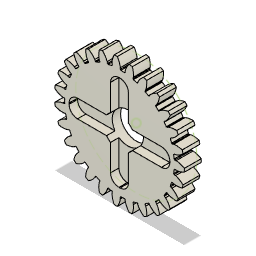
spurGearMaking (Autodesk Fusion 360 design; units mm, degrees)
description: Spur Gear; Module: 0.8; Num Teeth: 27; Pressure Angle: 20.0; Backlash: 0.00 mm
Autodesk Fusion 360 part; units mm, degrees
(part 1 of 3)
sketch "Sketch1" plane through (0, 0, 0) normal (0, 0, 1) x (1, 0, 0) in component "Spur Gear (27 teeth)"
  circle A0 centre (0, 0) radius 9.7892
  circle A1 centre (0, 0) radius 2.8
extrude "Extrude1" add sketch "Sketch1" along normal blind 3 in component "Spur Gear (27 teeth)"
sketch "Sketch2" plane through (0, 0, 0) normal (0, 0, 1) x (1, 0, 0) in component "Spur Gear (27 teeth)"
  spline S0 degree 5 poles (10.1216, -0.741) (10.1258, -0.7413) (10.1342, -0.7418) (10.1468, -0.7423) (10.1637, -0.7423) (10.1848, -0.7416) (10.2059, -0.7403) (10.2271, -0.7386) (10.2482, -0.7368) (10.2694, -0.7348) (10.2906, -0.7326) (10.3117, -0.7303) (10.3329, -0.7277) (10.3541, -0.7249) (10.3753, -0.7218) (10.3965, -0.7184) (10.4177, -0.7149) (10.4389, -0.7111) (10.4601, -0.7072) (10.4813, -0.7031) (10.5025, -0.6988) (10.5237, -0.6944) (10.5449, -0.6898) (10.5661, -0.6851) (10.5874, -0.6802) (10.6086, -0.6751) (10.6297, -0.6698) (10.6509, -0.6645) (10.6721, -0.6589) (10.6933, -0.6532) (10.7145, -0.6474) (10.7357, -0.6415) (10.7569, -0.6353) (10.778, -0.6291) (10.7992, -0.6227) (10.8204, -0.6162) (10.8415, -0.6096) (10.8627, -0.6028) (10.8838, -0.5959) (10.9049, -0.5888) (10.926, -0.5817) (10.9472, -0.5744) (10.9683, -0.5669) (10.9894, -0.5594) (11.0105, -0.5517) (11.0315, -0.544) (11.0526, -0.536) (11.0737, -0.528) (11.0947, -0.5199) (11.1158, -0.5116) (11.1368, -0.5032) (11.1578, -0.4947) (11.1788, -0.4861) (11.1998, -0.4774) (11.2208, -0.4686) (11.2418, -0.4596) (11.2628, -0.4506) (11.2837, -0.4414) (11.3047, -0.4321) (11.3256, -0.4227) (11.3465, -0.4132) (11.3674, -0.4036) (11.3883, -0.3939) (11.4092, -0.3841) (11.43, -0.3742) (11.4509, -0.3641) (11.4717, -0.354) (11.4925, -0.3438) (11.5133, -0.3334) (11.5341, -0.323) (11.5549, -0.3124) (11.5715, -0.3039) (11.5839, -0.2975) (11.5922, -0.2931) (11.5963, -0.291) knots 0 0 0 0 0 0 0.01428571 0.02857143 0.04285714 0.05714286 0.07142857 0.08571429 0.1 0.11428571 0.12857143 0.14285714 0.15714286 0.17142857 0.18571429 0.2 0.21428571 0.22857143 0.24285714 0.25714286 0.27142857 0.28571429 0.3 0.31428571 0.32857143 0.34285714 0.35714286 0.37142857 0.38571429 0.4 0.41428571 0.42857143 0.44285714 0.45714286 0.47142857 0.48571429 0.5 0.51428571 0.52857143 0.54285714 0.55714286 0.57142857 0.58571429 0.6 0.61428571 0.62857143 0.64285714 0.65714286 0.67142857 0.68571429 0.7 0.71428571 0.72857143 0.74285714 0.75714286 0.77142857 0.78571429 0.8 0.81428571 0.82857143 0.84285714 0.85714286 0.87142857 0.88571429 0.9 0.91428571 0.92857143 0.94285714 0.95714286 0.97142857 0.98571429 1 1 1 1 1 1
  spline S1 degree 5 poles (10.1216, 0.741) (10.1258, 0.7413) (10.1342, 0.7418) (10.1468, 0.7423) (10.1637, 0.7423) (10.1848, 0.7416) (10.2059, 0.7403) (10.2271, 0.7386) (10.2482, 0.7368) (10.2694, 0.7348) (10.2906, 0.7326) (10.3117, 0.7303) (10.3329, 0.7277) (10.3541, 0.7249) (10.3753, 0.7218) (10.3965, 0.7184) (10.4177, 0.7149) (10.4389, 0.7111) (10.4601, 0.7072) (10.4813, 0.7031) (10.5025, 0.6988) (10.5237, 0.6944) (10.5449, 0.6898) (10.5661, 0.6851) (10.5874, 0.6802) (10.6086, 0.6751) (10.6297, 0.6698) (10.6509, 0.6645) (10.6721, 0.6589) (10.6933, 0.6532) (10.7145, 0.6474) (10.7357, 0.6415) (10.7569, 0.6353) (10.778, 0.6291) (10.7992, 0.6227) (10.8204, 0.6162) (10.8415, 0.6096) (10.8627, 0.6028) (10.8838, 0.5959) (10.9049, 0.5888) (10.926, 0.5817) (10.9472, 0.5744) (10.9683, 0.5669) (10.9894, 0.5594) (11.0105, 0.5517) (11.0315, 0.544) (11.0526, 0.536) (11.0737, 0.528) (11.0947, 0.5199) (11.1158, 0.5116) (11.1368, 0.5032) (11.1578, 0.4947) (11.1788, 0.4861) (11.1998, 0.4774) (11.2208, 0.4686) (11.2418, 0.4596) (11.2628, 0.4506) (11.2837, 0.4414) (11.3047, 0.4321) (11.3256, 0.4227) (11.3465, 0.4132) (11.3674, 0.4036) (11.3883, 0.3939) (11.4092, 0.3841) (11.43, 0.3742) (11.4509, 0.3641) (11.4717, 0.354) (11.4925, 0.3438) (11.5133, 0.3334) (11.5341, 0.323) (11.5549, 0.3124) (11.5715, 0.3039) (11.5839, 0.2975) (11.5922, 0.2931) (11.5963, 0.291) knots 0 0 0 0 0 0 0.01428571 0.02857143 0.04285714 0.05714286 0.07142857 0.08571429 0.1 0.11428571 0.12857143 0.14285714 0.15714286 0.17142857 0.18571429 0.2 0.21428571 0.22857143 0.24285714 0.25714286 0.27142857 0.28571429 0.3 0.31428571 0.32857143 0.34285714 0.35714286 0.37142857 0.38571429 0.4 0.41428571 0.42857143 0.44285714 0.45714286 0.47142857 0.48571429 0.5 0.51428571 0.52857143 0.54285714 0.55714286 0.57142857 0.58571429 0.6 0.61428571 0.62857143 0.64285714 0.65714286 0.67142857 0.68571429 0.7 0.71428571 0.72857143 0.74285714 0.75714286 0.77142857 0.78571429 0.8 0.81428571 0.82857143 0.84285714 0.85714286 0.87142857 0.88571429 0.9 0.91428571 0.92857143 0.94285714 0.95714286 0.97142857 0.98571429 1 1 1 1 1 1
  arc A0 (11.5963, -0.291) -> (11.5963, 0.291) centre (0, 0) ccw
  line L0 (9.7531, -0.7148) -> (10.1216, -0.741)
  line L1 (9.7531, 0.7148) -> (10.1216, 0.741)
  line L2 (9.7531, -0.7148) -> (9.7531, 0.7148)
  point P0 (10.2257, -0.7387)
  point P1 (10.3304, -0.728)
  point P2 (10.4354, -0.7117)
  point P3 (10.5407, -0.6907)
  point P4 (10.6462, -0.6656)
  point P5 (10.7518, -0.6368)
  point P6 (10.8575, -0.6044)
  point P7 (10.9633, -0.5687)
  point P8 (11.069, -0.5298)
  point P9 (11.1747, -0.4878)
  point P10 (11.2803, -0.4429)
  point P11 (11.3858, -0.395)
  point P12 (11.4912, -0.3444)
  point P13 (10.2257, 0.7387)
  point P14 (10.3304, 0.728)
  point P15 (10.4354, 0.7117)
  point P16 (10.5407, 0.6907)
  point P17 (10.6462, 0.6656)
  point P18 (10.7518, 0.6368)
  point P19 (10.8575, 0.6044)
  point P20 (10.9633, 0.5687)
  point P21 (11.069, 0.5298)
  point P22 (11.1747, 0.4878)
  point P23 (11.2803, 0.4429)
  point P24 (11.3858, 0.395)
  point P25 (11.4912, 0.3444)
extrude "Extrude2" add sketch "Sketch2" along normal blind 3 in component "Spur Gear (27 teeth)"
fillet "Fillet1" radius 0.1 2 edges at (9.763, -0.7155, 1.5) (9.763, 0.7155, 1.5) in component "Spur Gear (27 teeth)"
pattern_circular "C-Pattern1" count 27 over 360 about axis through (0, 0, 0) along (0, 0, 1) of "Extrude2", "Fillet1" in component "Spur Gear (27 teeth)"
sketch "Sketch3" plane through (0, 0, 0) normal (0, 0, 1) x (1, 0, 0) in component "Spur Gear (27 teeth)"
  circle A0 centre (0, 0) radius 10.8 construction
sketch "Sketch4" plane through (0, 0, 3) normal (0, 0, 1) x (1, 0, 0) in component "Spur Gear (27 teeth)"
  arc A0 (9.6801, -1.4577) -> (9.7553, -0.814) centre (0, 0) ccw
  arc A1 (9.8621, -0.7225) -> (9.7553, -0.814) centre (9.855, -0.8223) ccw
  line L0 (9.8621, -0.7225) -> (10.1216, -0.741)
  spline S0 degree 5 poles (10.1216, -0.741) (10.1258, -0.7413) (10.1342, -0.7418) (10.1468, -0.7423) (10.1637, -0.7423) (10.1848, -0.7416) (10.2059, -0.7403) (10.2271, -0.7386) (10.2482, -0.7368) (10.2694, -0.7348) (10.2906, -0.7326) (10.3117, -0.7303) (10.3329, -0.7277) (10.3541, -0.7249) (10.3753, -0.7218) (10.3965, -0.7184) (10.4177, -0.7149) (10.4389, -0.7111) (10.4601, -0.7072) (10.4813, -0.7031) (10.5025, -0.6988) (10.5237, -0.6944) (10.5449, -0.6898) (10.5661, -0.6851) (10.5874, -0.6802) (10.6086, -0.6751) (10.6297, -0.6698) (10.6509, -0.6645) (10.6721, -0.6589) (10.6933, -0.6532) (10.7145, -0.6474) (10.7357, -0.6415) (10.7569, -0.6353) (10.778, -0.6291) (10.7992, -0.6227) (10.8204, -0.6162) (10.8415, -0.6096) (10.8627, -0.6028) (10.8838, -0.5959) (10.9049, -0.5888) (10.926, -0.5817) (10.9472, -0.5744) (10.9683, -0.5669) (10.9894, -0.5594) (11.0105, -0.5517) (11.0315, -0.544) (11.0526, -0.536) (11.0737, -0.528) (11.0947, -0.5199) (11.1158, -0.5116) (11.1368, -0.5032) (11.1578, -0.4947) (11.1788, -0.4861) (11.1998, -0.4774) (11.2208, -0.4686) (11.2418, -0.4596) (11.2628, -0.4506) (11.2837, -0.4414) (11.3047, -0.4321) (11.3256, -0.4227) (11.3465, -0.4132) (11.3674, -0.4036) (11.3883, -0.3939) (11.4092, -0.3841) (11.43, -0.3742) (11.4509, -0.3641) (11.4717, -0.354) (11.4925, -0.3438) (11.5133, -0.3334) (11.5341, -0.323) (11.5549, -0.3124) (11.5715, -0.3039) (11.5839, -0.2975) (11.5922, -0.2931) (11.5963, -0.291) knots 0 0 0 0 0 0 0.01428571 0.02857143 0.04285714 0.05714286 0.07142857 0.08571429 0.1 0.11428571 0.12857143 0.14285714 0.15714286 0.17142857 0.18571429 0.2 0.21428571 0.22857143 0.24285714 0.25714286 0.27142857 0.28571429 0.3 0.31428571 0.32857143 0.34285714 0.35714286 0.37142857 0.38571429 0.4 0.41428571 0.42857143 0.44285714 0.45714286 0.47142857 0.48571429 0.5 0.51428571 0.52857143 0.54285714 0.55714286 0.57142857 0.58571429 0.6 0.61428571 0.62857143 0.64285714 0.65714286 0.67142857 0.68571429 0.7 0.71428571 0.72857143 0.74285714 0.75714286 0.77142857 0.78571429 0.8 0.81428571 0.82857143 0.84285714 0.85714286 0.87142857 0.88571429 0.9 0.91428571 0.92857143 0.94285714 0.95714286 0.97142857 0.98571429 1 1 1 1 1 1
  arc A2 (11.5963, -0.291) -> (11.5963, 0.291) centre (0, 0) ccw
  spline S1 degree 5 poles (11.5963, 0.291) (11.5922, 0.2931) (11.5839, 0.2975) (11.5715, 0.3039) (11.5549, 0.3124) (11.5341, 0.323) (11.5133, 0.3334) (11.4925, 0.3438) (11.4717, 0.354) (11.4509, 0.3641) (11.43, 0.3742) (11.4092, 0.3841) (11.3883, 0.3939) (11.3674, 0.4036) (11.3465, 0.4132) (11.3256, 0.4227) (11.3047, 0.4321) (11.2837, 0.4414) (11.2628, 0.4506) (11.2418, 0.4596) (11.2208, 0.4686) (11.1998, 0.4774) (11.1788, 0.4861) (11.1578, 0.4947) (11.1368, 0.5032) (11.1158, 0.5116) (11.0947, 0.5199) (11.0737, 0.528) (11.0526, 0.536) (11.0315, 0.544) (11.0105, 0.5517) (10.9894, 0.5594) (10.9683, 0.5669) (10.9472, 0.5744) (10.926, 0.5817) (10.9049, 0.5888) (10.8838, 0.5959) (10.8627, 0.6028) (10.8415, 0.6096) (10.8204, 0.6162) (10.7992, 0.6227) (10.778, 0.6291) (10.7569, 0.6353) (10.7357, 0.6415) (10.7145, 0.6474) (10.6933, 0.6532) (10.6721, 0.6589) (10.6509, 0.6645) (10.6297, 0.6698) (10.6086, 0.6751) (10.5874, 0.6802) (10.5661, 0.6851) (10.5449, 0.6898) (10.5237, 0.6944) (10.5025, 0.6988) (10.4813, 0.7031) (10.4601, 0.7072) (10.4389, 0.7111) (10.4177, 0.7149) (10.3965, 0.7184) (10.3753, 0.7218) (10.3541, 0.7249) (10.3329, 0.7277) (10.3117, 0.7303) (10.2906, 0.7326) (10.2694, 0.7348) (10.2482, 0.7368) (10.2271, 0.7386) (10.2059, 0.7403) (10.1848, 0.7416) (10.1637, 0.7423) (10.1468, 0.7423) (10.1342, 0.7418) (10.1258, 0.7413) (10.1216, 0.741) knots -1 -1 -1 -1 -1 -1 -0.98571429 -0.97142857 -0.95714286 -0.94285714 -0.92857143 -0.91428571 -0.9 -0.88571429 -0.87142857 -0.85714286 -0.84285714 -0.82857143 -0.81428571 -0.8 -0.78571429 -0.77142857 -0.75714286 -0.74285714 -0.72857143 -0.71428571 -0.7 -0.68571429 -0.67142857 -0.65714286 -0.64285714 -0.62857143 -0.61428571 -0.6 -0.58571429 -0.57142857 -0.55714286 -0.54285714 -0.52857143 -0.51428571 -0.5 -0.48571429 -0.47142857 -0.45714286 -0.44285714 -0.42857143 -0.41428571 -0.4 -0.38571429 -0.37142857 -0.35714286 -0.34285714 -0.32857143 -0.31428571 -0.3 -0.28571429 -0.27142857 -0.25714286 -0.24285714 -0.22857143 -0.21428571 -0.2 -0.18571429 -0.17142857 -0.15714286 -0.14285714 -0.12857143 -0.11428571 -0.1 -0.08571429 -0.07142857 -0.05714286 -0.04285714 -0.02857143 -0.01428571 0 0 0 0 0 0
  line L1 (10.1216, 0.741) -> (9.8621, 0.7225)
  arc A3 (9.7553, 0.814) -> (9.8621, 0.7225) centre (9.855, 0.8223) ccw
  arc A4 (9.7553, 0.814) -> (9.6801, 1.4577) centre (0, 0) ccw
  arc A5 (9.7629, 1.5713) -> (9.6801, 1.4577) centre (9.7789, 1.4726) ccw
  line L2 (9.7629, 1.5713) -> (10.0197, 1.6131)
  spline S2 degree 5 poles (10.0197, 1.6131) (10.0238, 1.6138) (10.0321, 1.6153) (10.0445, 1.6178) (10.0609, 1.6216) (10.0813, 1.6272) (10.1016, 1.6333) (10.1217, 1.6398) (10.1419, 1.6465) (10.162, 1.6533) (10.1821, 1.6603) (10.2022, 1.6674) (10.2222, 1.6748) (10.2422, 1.6825) (10.2621, 1.6904) (10.282, 1.6985) (10.3018, 1.7069) (10.3215, 1.7155) (10.3412, 1.7242) (10.3609, 1.7331) (10.3806, 1.7421) (10.4002, 1.7512) (10.4198, 1.7606) (10.4393, 1.7701) (10.4588, 1.7798) (10.4783, 1.7896) (10.4977, 1.7996) (10.5171, 1.8097) (10.5364, 1.82) (10.5557, 1.8304) (10.575, 1.841) (10.5942, 1.8517) (10.6134, 1.8625) (10.6326, 1.8734) (10.6517, 1.8845) (10.6708, 1.8957) (10.6898, 1.9071) (10.7089, 1.9186) (10.7278, 1.9302) (10.7468, 1.9419) (10.7657, 1.9537) (10.7845, 1.9657) (10.8034, 1.9778) (10.8222, 1.99) (10.8409, 2.0023) (10.8596, 2.0148) (10.8783, 2.0273) (10.897, 2.04) (10.9156, 2.0528) (10.9341, 2.0657) (10.9527, 2.0787) (10.9712, 2.0918) (10.9896, 2.105) (11.008, 2.1183) (11.0264, 2.1318) (11.0448, 2.1453) (11.0631, 2.1589) (11.0814, 2.1727) (11.0996, 2.1866) (11.1178, 2.2005) (11.136, 2.2146) (11.1541, 2.2288) (11.1722, 2.243) (11.1902, 2.2574) (11.2082, 2.2719) (11.2262, 2.2864) (11.2441, 2.3011) (11.262, 2.3159) (11.2799, 2.3307) (11.2977, 2.3457) (11.3154, 2.3607) (11.3296, 2.3729) (11.3403, 2.382) (11.3473, 2.3881) (11.3509, 2.3912) knots 0 0 0 0 0 0 0.01428571 0.02857143 0.04285714 0.05714286 0.07142857 0.08571429 0.1 0.11428571 0.12857143 0.14285714 0.15714286 0.17142857 0.18571429 0.2 0.21428571 0.22857143 0.24285714 0.25714286 0.27142857 0.28571429 0.3 0.31428571 0.32857143 0.34285714 0.35714286 0.37142857 0.38571429 0.4 0.41428571 0.42857143 0.44285714 0.45714286 0.47142857 0.48571429 0.5 0.51428571 0.52857143 0.54285714 0.55714286 0.57142857 0.58571429 0.6 0.61428571 0.62857143 0.64285714 0.65714286 0.67142857 0.68571429 0.7 0.71428571 0.72857143 0.74285714 0.75714286 0.77142857 0.78571429 0.8 0.81428571 0.82857143 0.84285714 0.85714286 0.87142857 0.88571429 0.9 0.91428571 0.92857143 0.94285714 0.95714286 0.97142857 0.98571429 1 1 1 1 1 1
  arc A6 (11.3509, 2.3912) -> (11.2167, 2.9574) centre (0, 0) ccw
  spline S3 degree 5 poles (11.2167, 2.9574) (11.2121, 2.9586) (11.2031, 2.9609) (11.1895, 2.9643) (11.1714, 2.9687) (11.1487, 2.9742) (11.1261, 2.9796) (11.1035, 2.9848) (11.0808, 2.99) (11.0582, 2.9951) (11.0356, 3) (11.013, 3.0049) (10.9905, 3.0096) (10.9679, 3.0142) (10.9454, 3.0188) (10.9228, 3.0232) (10.9003, 3.0275) (10.8778, 3.0317) (10.8553, 3.0358) (10.8328, 3.0398) (10.8103, 3.0436) (10.7878, 3.0474) (10.7654, 3.051) (10.743, 3.0546) (10.7206, 3.058) (10.6982, 3.0613) (10.6758, 3.0645) (10.6534, 3.0676) (10.6311, 3.0705) (10.6087, 3.0733) (10.5864, 3.0761) (10.5641, 3.0786) (10.5419, 3.0811) (10.5196, 3.0835) (10.4974, 3.0857) (10.4752, 3.0878) (10.453, 3.0898) (10.4308, 3.0916) (10.4087, 3.0934) (10.3866, 3.0949) (10.3645, 3.0964) (10.3424, 3.0977) (10.3204, 3.0989) (10.2984, 3.1) (10.2764, 3.1009) (10.2544, 3.1017) (10.2325, 3.1023) (10.2106, 3.1028) (10.1887, 3.1032) (10.1669, 3.1034) (10.1451, 3.1035) (10.1233, 3.1033) (10.1016, 3.1031) (10.0799, 3.1026) (10.0583, 3.102) (10.0367, 3.1013) (10.0151, 3.1004) (9.9935, 3.0993) (9.972, 3.0981) (9.9506, 3.0967) (9.9292, 3.0951) (9.9078, 3.0932) (9.8866, 3.0911) (9.8654, 3.0887) (9.8442, 3.086) (9.8231, 3.0832) (9.8021, 3.0803) (9.7811, 3.0772) (9.7601, 3.074) (9.7393, 3.0704) (9.7186, 3.0662) (9.7022, 3.0623) (9.69, 3.0589) (9.6819, 3.0565) (9.6779, 3.0553) knots -1 -1 -1 -1 -1 -1 -0.98571429 -0.97142857 -0.95714286 -0.94285714 -0.92857143 -0.91428571 -0.9 -0.88571429 -0.87142857 -0.85714286 -0.84285714 -0.82857143 -0.81428571 -0.8 -0.78571429 -0.77142857 -0.75714286 -0.74285714 -0.72857143 -0.71428571 -0.7 -0.68571429 -0.67142857 -0.65714286 -0.64285714 -0.62857143 -0.61428571 -0.6 -0.58571429 -0.57142857 -0.55714286 -0.54285714 -0.52857143 -0.51428571 -0.5 -0.48571429 -0.47142857 -0.45714286 -0.44285714 -0.42857143 -0.41428571 -0.4 -0.38571429 -0.37142857 -0.35714286 -0.34285714 -0.32857143 -0.31428571 -0.3 -0.28571429 -0.27142857 -0.25714286 -0.24285714 -0.22857143 -0.21428571 -0.2 -0.18571429 -0.17142857 -0.15714286 -0.14285714 -0.12857143 -0.11428571 -0.1 -0.08571429 -0.07142857 -0.05714286 -0.04285714 -0.02857143 -0.01428571 0 0 0 0 0 0
  line L3 (9.6779, 3.0553) -> (9.4296, 2.9774)
  arc A7 (9.3046, 3.0418) -> (9.4296, 2.9774) centre (9.3997, 3.0728) ccw
  arc A8 (9.3046, 3.0418) -> (9.083, 3.6508) centre (0, 0) ccw
  arc A9 (9.1373, 3.7804) -> (9.083, 3.6508) centre (9.1758, 3.6881) ccw
  line L4 (9.1373, 3.7804) -> (9.3776, 3.8804)
  spline S4 degree 5 poles (9.3776, 3.8804) (9.3814, 3.882) (9.3892, 3.8853) (9.4007, 3.8906) (9.4158, 3.8981) (9.4343, 3.9082) (9.4526, 3.9189) (9.4707, 3.9298) (9.4888, 3.941) (9.5068, 3.9523) (9.5248, 3.9637) (9.5427, 3.9753) (9.5604, 3.9871) (9.5781, 3.9991) (9.5957, 4.0114) (9.6131, 4.0239) (9.6304, 4.0366) (9.6477, 4.0495) (9.6649, 4.0626) (9.682, 4.0757) (9.699, 4.089) (9.716, 4.1025) (9.7329, 4.1161) (9.7497, 4.1299) (9.7665, 4.1438) (9.7831, 4.1578) (9.7997, 4.172) (9.8162, 4.1864) (9.8327, 4.2008) (9.8491, 4.2154) (9.8654, 4.2301) (9.8816, 4.2449) (9.8978, 4.2599) (9.9139, 4.275) (9.93, 4.2902) (9.946, 4.3055) (9.9619, 4.3209) (9.9777, 4.3365) (9.9935, 4.3522) (10.0093, 4.3679) (10.0249, 4.3838) (10.0405, 4.3998) (10.0561, 4.4159) (10.0715, 4.4321) (10.0869, 4.4484) (10.1023, 4.4649) (10.1176, 4.4814) (10.1328, 4.498) (10.1479, 4.5147) (10.163, 4.5316) (10.1781, 4.5485) (10.193, 4.5655) (10.208, 4.5826) (10.2228, 4.5998) (10.2376, 4.6172) (10.2523, 4.6346) (10.267, 4.6521) (10.2816, 4.6697) (10.2961, 4.6874) (10.3106, 4.7051) (10.3251, 4.723) (10.3394, 4.741) (10.3537, 4.759) (10.368, 4.7772) (10.3822, 4.7954) (10.3963, 4.8137) (10.4104, 4.8321) (10.4244, 4.8506) (10.4383, 4.8692) (10.4522, 4.8879) (10.466, 4.9066) (10.477, 4.9217) (10.4853, 4.933) (10.4907, 4.9406) (10.4935, 4.9444) knots 0 0 0 0 0 0 0.01428571 0.02857143 0.04285714 0.05714286 0.07142857 0.08571429 0.1 0.11428571 0.12857143 0.14285714 0.15714286 0.17142857 0.18571429 0.2 0.21428571 0.22857143 0.24285714 0.25714286 0.27142857 0.28571429 0.3 0.31428571 0.32857143 0.34285714 0.35714286 0.37142857 0.38571429 0.4 0.41428571 0.42857143 0.44285714 0.45714286 0.47142857 0.48571429 0.5 0.51428571 0.52857143 0.54285714 0.55714286 0.57142857 0.58571429 0.6 0.61428571 0.62857143 0.64285714 0.65714286 0.67142857 0.68571429 0.7 0.71428571 0.72857143 0.74285714 0.75714286 0.77142857 0.78571429 0.8 0.81428571 0.82857143 0.84285714 0.85714286 0.87142857 0.88571429 0.9 0.91428571 0.92857143 0.94285714 0.95714286 0.97142857 0.98571429 1 1 1 1 1 1
  arc A10 (10.4935, 4.9444) -> (10.2323, 5.4645) centre (0, 0) ccw
  spline S5 degree 5 poles (10.2323, 5.4645) (10.2276, 5.4645) (10.2183, 5.4647) (10.2043, 5.4648) (10.1856, 5.465) (10.1623, 5.4651) (10.139, 5.4651) (10.1158, 5.465) (10.0926, 5.4648) (10.0694, 5.4645) (10.0463, 5.4642) (10.0232, 5.4637) (10.0002, 5.4631) (9.9771, 5.4624) (9.9541, 5.4616) (9.9312, 5.4607) (9.9083, 5.4597) (9.8854, 5.4586) (9.8626, 5.4574) (9.8398, 5.4561) (9.817, 5.4546) (9.7943, 5.4531) (9.7716, 5.4515) (9.749, 5.4497) (9.7264, 5.4479) (9.7038, 5.4459) (9.6813, 5.4439) (9.6588, 5.4417) (9.6364, 5.4394) (9.614, 5.437) (9.5917, 5.4345) (9.5694, 5.4319) (9.5472, 5.4292) (9.525, 5.4263) (9.5028, 5.4234) (9.4807, 5.4203) (9.4587, 5.4171) (9.4367, 5.4138) (9.4148, 5.4104) (9.3929, 5.4068) (9.371, 5.4032) (9.3493, 5.3994) (9.3275, 5.3954) (9.3059, 5.3914) (9.2843, 5.3872) (9.2627, 5.3829) (9.2413, 5.3785) (9.2198, 5.3739) (9.1985, 5.3692) (9.1772, 5.3644) (9.1559, 5.3594) (9.1348, 5.3543) (9.1137, 5.349) (9.0927, 5.3436) (9.0718, 5.338) (9.0509, 5.3323) (9.0301, 5.3264) (9.0094, 5.3204) (8.9888, 5.3143) (8.9682, 5.308) (8.9478, 5.3015) (8.9274, 5.2947) (8.9072, 5.2877) (8.8872, 5.2805) (8.8672, 5.2731) (8.8473, 5.2655) (8.8275, 5.2578) (8.8077, 5.25) (8.7881, 5.242) (8.7687, 5.2336) (8.7495, 5.2248) (8.7344, 5.2172) (8.7233, 5.2111) (8.716, 5.2069) (8.7124, 5.2048) knots -1 -1 -1 -1 -1 -1 -0.98571429 -0.97142857 -0.95714286 -0.94285714 -0.92857143 -0.91428571 -0.9 -0.88571429 -0.87142857 -0.85714286 -0.84285714 -0.82857143 -0.81428571 -0.8 -0.78571429 -0.77142857 -0.75714286 -0.74285714 -0.72857143 -0.71428571 -0.7 -0.68571429 -0.67142857 -0.65714286 -0.64285714 -0.62857143 -0.61428571 -0.6 -0.58571429 -0.57142857 -0.55714286 -0.54285714 -0.52857143 -0.51428571 -0.5 -0.48571429 -0.47142857 -0.45714286 -0.44285714 -0.42857143 -0.41428571 -0.4 -0.38571429 -0.37142857 -0.35714286 -0.34285714 -0.32857143 -0.31428571 -0.3 -0.28571429 -0.27142857 -0.25714286 -0.24285714 -0.22857143 -0.21428571 -0.2 -0.18571429 -0.17142857 -0.15714286 -0.14285714 -0.12857143 -0.11428571 -0.1 -0.08571429 -0.07142857 -0.05714286 -0.04285714 -0.02857143 -0.01428571 0 0 0 0 0 0
  line L5 (8.7124, 5.2048) -> (8.4888, 5.0718)
  arc A11 (8.3523, 5.1056) -> (8.4888, 5.0718) centre (8.4377, 5.1577) ccw
  arc A12 (8.3523, 5.1056) -> (7.9962, 5.647) centre (0, 0) ccw
  arc A13 (8.0192, 5.7857) -> (7.9962, 5.647) centre (8.0779, 5.7047) ccw
  line L6 (8.0192, 5.7857) -> (8.2299, 5.9384)
  spline S6 degree 5 poles (8.2299, 5.9384) (8.2333, 5.9408) (8.2401, 5.9459) (8.2501, 5.9536) (8.263, 5.9645) (8.2787, 5.9786) (8.294, 5.9932) (8.3092, 6.008) (8.3242, 6.023) (8.3391, 6.0382) (8.3539, 6.0534) (8.3687, 6.0688) (8.3833, 6.0844) (8.3977, 6.1002) (8.4119, 6.1162) (8.426, 6.1324) (8.4399, 6.1488) (8.4537, 6.1653) (8.4675, 6.1819) (8.4811, 6.1987) (8.4946, 6.2156) (8.508, 6.2326) (8.5213, 6.2497) (8.5345, 6.267) (8.5476, 6.2844) (8.5606, 6.3019) (8.5734, 6.3195) (8.5862, 6.3373) (8.5989, 6.3552) (8.6115, 6.3731) (8.6239, 6.3912) (8.6363, 6.4094) (8.6486, 6.4277) (8.6608, 6.4461) (8.6729, 6.4646) (8.685, 6.4831) (8.6969, 6.5018) (8.7087, 6.5206) (8.7205, 6.5395) (8.7321, 6.5585) (8.7437, 6.5776) (8.7552, 6.5967) (8.7666, 6.616) (8.7779, 6.6353) (8.7892, 6.6547) (8.8003, 6.6742) (8.8114, 6.6939) (8.8223, 6.7135) (8.8332, 6.7333) (8.844, 6.7532) (8.8548, 6.7731) (8.8654, 6.7931) (8.876, 6.8132) (8.8865, 6.8334) (8.8968, 6.8537) (8.9072, 6.874) (8.9174, 6.8944) (8.9276, 6.9149) (8.9376, 6.9355) (8.9476, 6.9561) (8.9575, 6.9768) (8.9674, 6.9976) (8.9771, 7.0185) (8.9868, 7.0394) (8.9964, 7.0604) (9.0059, 7.0815) (9.0154, 7.1027) (9.0247, 7.1239) (9.034, 7.1452) (9.0432, 7.1666) (9.0524, 7.188) (9.0596, 7.2052) (9.065, 7.2181) (9.0686, 7.2268) (9.0704, 7.2311) knots 0 0 0 0 0 0 0.01428571 0.02857143 0.04285714 0.05714286 0.07142857 0.08571429 0.1 0.11428571 0.12857143 0.14285714 0.15714286 0.17142857 0.18571429 0.2 0.21428571 0.22857143 0.24285714 0.25714286 0.27142857 0.28571429 0.3 0.31428571 0.32857143 0.34285714 0.35714286 0.37142857 0.38571429 0.4 0.41428571 0.42857143 0.44285714 0.45714286 0.47142857 0.48571429 0.5 0.51428571 0.52857143 0.54285714 0.55714286 0.57142857 0.58571429 0.6 0.61428571 0.62857143 0.64285714 0.65714286 0.67142857 0.68571429 0.7 0.71428571 0.72857143 0.74285714 0.75714286 0.77142857 0.78571429 0.8 0.81428571 0.82857143 0.84285714 0.85714286 0.87142857 0.88571429 0.9 0.91428571 0.92857143 0.94285714 0.95714286 0.97142857 0.98571429 1 1 1 1 1 1
  arc A14 (9.0704, 7.2311) -> (8.6963, 7.6769) centre (0, 0) ccw
  spline S7 degree 5 poles (8.6963, 7.6769) (8.6917, 7.6759) (8.6826, 7.6739) (8.6689, 7.6708) (8.6507, 7.6666) (8.628, 7.6614) (8.6054, 7.656) (8.5828, 7.6506) (8.5603, 7.645) (8.5378, 7.6394) (8.5154, 7.6337) (8.493, 7.6279) (8.4707, 7.622) (8.4485, 7.616) (8.4263, 7.6099) (8.4042, 7.6038) (8.3821, 7.5975) (8.3601, 7.5912) (8.3382, 7.5847) (8.3163, 7.5782) (8.2945, 7.5716) (8.2727, 7.5648) (8.251, 7.558) (8.2294, 7.5511) (8.2078, 7.5441) (8.1863, 7.537) (8.1649, 7.5298) (8.1435, 7.5225) (8.1222, 7.5151) (8.101, 7.5076) (8.0799, 7.5) (8.0588, 7.4924) (8.0378, 7.4846) (8.0168, 7.4767) (7.996, 7.4687) (7.9752, 7.4606) (7.9545, 7.4524) (7.9338, 7.4441) (7.9133, 7.4357) (7.8928, 7.4272) (7.8724, 7.4186) (7.8521, 7.4099) (7.8318, 7.4011) (7.8117, 7.3921) (7.7916, 7.3831) (7.7717, 7.3739) (7.7518, 7.3647) (7.732, 7.3553) (7.7123, 7.3458) (7.6927, 7.3362) (7.6732, 7.3265) (7.6538, 7.3166) (7.6345, 7.3066) (7.6153, 7.2965) (7.5962, 7.2862) (7.5772, 7.2758) (7.5584, 7.2653) (7.5396, 7.2547) (7.5209, 7.244) (7.5024, 7.2331) (7.484, 7.2221) (7.4657, 7.2108) (7.4477, 7.1994) (7.4298, 7.1877) (7.4121, 7.1759) (7.3945, 7.1639) (7.377, 7.1518) (7.3596, 7.1397) (7.3423, 7.1273) (7.3253, 7.1148) (7.3087, 7.1018) (7.2958, 7.0909) (7.2864, 7.0824) (7.2803, 7.0766) (7.2773, 7.0737) knots -1 -1 -1 -1 -1 -1 -0.98571429 -0.97142857 -0.95714286 -0.94285714 -0.92857143 -0.91428571 -0.9 -0.88571429 -0.87142857 -0.85714286 -0.84285714 -0.82857143 -0.81428571 -0.8 -0.78571429 -0.77142857 -0.75714286 -0.74285714 -0.72857143 -0.71428571 -0.7 -0.68571429 -0.67142857 -0.65714286 -0.64285714 -0.62857143 -0.61428571 -0.6 -0.58571429 -0.57142857 -0.55714286 -0.54285714 -0.52857143 -0.51428571 -0.5 -0.48571429 -0.47142857 -0.45714286 -0.44285714 -0.42857143 -0.41428571 -0.4 -0.38571429 -0.37142857 -0.35714286 -0.34285714 -0.32857143 -0.31428571 -0.3 -0.28571429 -0.27142857 -0.25714286 -0.24285714 -0.22857143 -0.21428571 -0.2 -0.18571429 -0.17142857 -0.15714286 -0.14285714 -0.12857143 -0.11428571 -0.1 -0.08571429 -0.07142857 -0.05714286 -0.04285714 -0.02857143 -0.01428571 0 0 0 0 0 0
  line L7 (7.2773, 7.0737) -> (7.0903, 6.8927)
  arc A15 (6.9498, 6.8941) -> (7.0903, 6.8927) centre (7.0208, 6.9646) ccw
  arc A16 (6.9498, 6.8941) -> (6.4784, 7.3389) centre (0, 0) ccw
  arc A17 (6.4688, 7.4791) -> (6.4784, 7.3389) centre (6.5445, 7.4139) ccw
  line L8 (6.4688, 7.4791) -> (6.6386, 7.6763)
  spline S8 degree 5 poles (6.6386, 7.6763) (6.6413, 7.6794) (6.6468, 7.6859) (6.6547, 7.6958) (6.6648, 7.7093) (6.6768, 7.7266) (6.6884, 7.7443) (6.6997, 7.7623) (6.7108, 7.7804) (6.7218, 7.7985) (6.7327, 7.8168) (6.7435, 7.8352) (6.7541, 7.8537) (6.7645, 7.8724) (6.7747, 7.8912) (6.7846, 7.9103) (6.7944, 7.9294) (6.8041, 7.9487) (6.8136, 7.968) (6.823, 7.9875) (6.8322, 8.007) (6.8413, 8.0267) (6.8503, 8.0464) (6.8592, 8.0662) (6.8679, 8.0862) (6.8765, 8.1062) (6.8849, 8.1264) (6.8933, 8.1466) (6.9015, 8.1669) (6.9096, 8.1873) (6.9176, 8.2077) (6.9254, 8.2283) (6.9332, 8.2489) (6.9408, 8.2696) (6.9483, 8.2904) (6.9557, 8.3113) (6.963, 8.3322) (6.9702, 8.3532) (6.9773, 8.3743) (6.9843, 8.3955) (6.9911, 8.4167) (6.9979, 8.438) (7.0046, 8.4594) (7.0111, 8.4808) (7.0176, 8.5023) (7.0239, 8.5238) (7.0301, 8.5455) (7.0363, 8.5671) (7.0423, 8.5889) (7.0483, 8.6107) (7.0541, 8.6326) (7.0598, 8.6545) (7.0655, 8.6765) (7.071, 8.6986) (7.0765, 8.7207) (7.0818, 8.7428) (7.0871, 8.7651) (7.0922, 8.7873) (7.0973, 8.8097) (7.1023, 8.8321) (7.1071, 8.8545) (7.1119, 8.877) (7.1166, 8.8996) (7.1212, 8.9222) (7.1257, 8.9448) (7.1301, 8.9676) (7.1344, 8.9903) (7.1386, 9.0131) (7.1427, 9.036) (7.1467, 9.0589) (7.1507, 9.0819) (7.1538, 9.1003) (7.156, 9.1141) (7.1575, 9.1233) (7.1583, 9.1279) knots 0 0 0 0 0 0 0.01428571 0.02857143 0.04285714 0.05714286 0.07142857 0.08571429 0.1 0.11428571 0.12857143 0.14285714 0.15714286 0.17142857 0.18571429 0.2 0.21428571 0.22857143 0.24285714 0.25714286 0.27142857 0.28571429 0.3 0.31428571 0.32857143 0.34285714 0.35714286 0.37142857 0.38571429 0.4 0.41428571 0.42857143 0.44285714 0.45714286 0.47142857 0.48571429 0.5 0.51428571 0.52857143 0.54285714 0.55714286 0.57142857 0.58571429 0.6 0.61428571 0.62857143 0.64285714 0.65714286 0.67142857 0.68571429 0.7 0.71428571 0.72857143 0.74285714 0.75714286 0.77142857 0.78571429 0.8 0.81428571 0.82857143 0.84285714 0.85714286 0.87142857 0.88571429 0.9 0.91428571 0.92857143 0.94285714 0.95714286 0.97142857 0.98571429 1 1 1 1 1 1
  arc A18 (7.1583, 9.1279) -> (6.6915, 9.4755) centre (0, 0) ccw
  spline S9 degree 5 poles (6.6915, 9.4755) (6.6872, 9.4734) (6.6788, 9.4694) (6.6662, 9.4632) (6.6495, 9.455) (6.6286, 9.4446) (6.6078, 9.4342) (6.5871, 9.4237) (6.5665, 9.4131) (6.5459, 9.4025) (6.5254, 9.3917) (6.505, 9.3809) (6.4846, 9.37) (6.4644, 9.3591) (6.4442, 9.3481) (6.4241, 9.337) (6.4041, 9.3258) (6.3841, 9.3145) (6.3642, 9.3032) (6.3445, 9.2918) (6.3248, 9.2803) (6.3051, 9.2687) (6.2856, 9.2571) (6.2662, 9.2454) (6.2468, 9.2336) (6.2275, 9.2217) (6.2083, 9.2098) (6.1892, 9.1978) (6.1702, 9.1857) (6.1513, 9.1735) (6.1324, 9.1612) (6.1137, 9.1489) (6.095, 9.1365) (6.0765, 9.124) (6.058, 9.1114) (6.0397, 9.0987) (6.0214, 9.086) (6.0032, 9.0731) (5.9852, 9.0602) (5.9672, 9.0472) (5.9493, 9.0342) (5.9316, 9.021) (5.9139, 9.0077) (5.8964, 8.9944) (5.879, 8.981) (5.8616, 8.9674) (5.8444, 8.9538) (5.8273, 8.9402) (5.8103, 8.9264) (5.7935, 8.9125) (5.7767, 8.8985) (5.7601, 8.8845) (5.7437, 8.8703) (5.7273, 8.856) (5.7111, 8.8416) (5.6951, 8.8272) (5.6791, 8.8126) (5.6633, 8.7979) (5.6476, 8.7832) (5.6321, 8.7683) (5.6167, 8.7533) (5.6016, 8.7382) (5.5867, 8.7228) (5.572, 8.7074) (5.5574, 8.6918) (5.5431, 8.6761) (5.5288, 8.6603) (5.5147, 8.6444) (5.5008, 8.6285) (5.4871, 8.6123) (5.4739, 8.5958) (5.4639, 8.5823) (5.4567, 8.5719) (5.4521, 8.5648) (5.4498, 8.5613) knots -1 -1 -1 -1 -1 -1 -0.98571429 -0.97142857 -0.95714286 -0.94285714 -0.92857143 -0.91428571 -0.9 -0.88571429 -0.87142857 -0.85714286 -0.84285714 -0.82857143 -0.81428571 -0.8 -0.78571429 -0.77142857 -0.75714286 -0.74285714 -0.72857143 -0.71428571 -0.7 -0.68571429 -0.67142857 -0.65714286 -0.64285714 -0.62857143 -0.61428571 -0.6 -0.58571429 -0.57142857 -0.55714286 -0.54285714 -0.52857143 -0.51428571 -0.5 -0.48571429 -0.47142857 -0.45714286 -0.44285714 -0.42857143 -0.41428571 -0.4 -0.38571429 -0.37142857 -0.35714286 -0.34285714 -0.32857143 -0.31428571 -0.3 -0.28571429 -0.27142857 -0.25714286 -0.24285714 -0.22857143 -0.21428571 -0.2 -0.18571429 -0.17142857 -0.15714286 -0.14285714 -0.12857143 -0.11428571 -0.1 -0.08571429 -0.07142857 -0.05714286 -0.04285714 -0.02857143 -0.01428571 0 0 0 0 0 0
  line L9 (5.4498, 8.5613) -> (5.3096, 8.3421)
  arc A19 (5.1726, 8.311) -> (5.3096, 8.3421) centre (5.2254, 8.3959) ccw
  arc A20 (5.1726, 8.311) -> (4.6113, 8.6351) centre (0, 0) ccw
  arc A21 (4.5696, 8.7693) -> (4.6113, 8.6351) centre (4.6584, 8.7233) ccw
  line L10 (4.5696, 8.7693) -> (4.6894, 9.0003)
  spline S10 degree 5 poles (4.6894, 9.0003) (4.6913, 9.004) (4.6951, 9.0116) (4.7005, 9.023) (4.7072, 9.0385) (4.7149, 9.0581) (4.7221, 9.078) (4.729, 9.0981) (4.7356, 9.1183) (4.7422, 9.1385) (4.7486, 9.1588) (4.7548, 9.1791) (4.7609, 9.1996) (4.7667, 9.2202) (4.7722, 9.2409) (4.7775, 9.2617) (4.7826, 9.2826) (4.7876, 9.3035) (4.7924, 9.3246) (4.797, 9.3457) (4.8015, 9.3668) (4.8059, 9.388) (4.8101, 9.4093) (4.8141, 9.4307) (4.818, 9.4521) (4.8217, 9.4736) (4.8253, 9.4951) (4.8287, 9.5167) (4.832, 9.5383) (4.8352, 9.5601) (4.8383, 9.5818) (4.8412, 9.6036) (4.844, 9.6255) (4.8466, 9.6474) (4.8491, 9.6693) (4.8515, 9.6914) (4.8538, 9.7134) (4.856, 9.7355) (4.858, 9.7577) (4.8599, 9.7799) (4.8617, 9.8021) (4.8633, 9.8244) (4.8649, 9.8467) (4.8663, 9.8691) (4.8676, 9.8915) (4.8688, 9.9139) (4.8699, 9.9364) (4.8709, 9.9589) (4.8718, 9.9815) (4.8725, 10.004) (4.8731, 10.0267) (4.8737, 10.0493) (4.8741, 10.072) (4.8744, 10.0948) (4.8746, 10.1176) (4.8747, 10.1404) (4.8747, 10.1632) (4.8746, 10.1861) (4.8743, 10.209) (4.874, 10.2319) (4.8736, 10.2549) (4.873, 10.2779) (4.8724, 10.3009) (4.8716, 10.3239) (4.8708, 10.347) (4.8698, 10.3701) (4.8688, 10.3933) (4.8676, 10.4165) (4.8663, 10.4396) (4.865, 10.4629) (4.8635, 10.4861) (4.8623, 10.5047) (4.8613, 10.5187) (4.8606, 10.528) (4.8603, 10.5327) knots 0 0 0 0 0 0 0.01428571 0.02857143 0.04285714 0.05714286 0.07142857 0.08571429 0.1 0.11428571 0.12857143 0.14285714 0.15714286 0.17142857 0.18571429 0.2 0.21428571 0.22857143 0.24285714 0.25714286 0.27142857 0.28571429 0.3 0.31428571 0.32857143 0.34285714 0.35714286 0.37142857 0.38571429 0.4 0.41428571 0.42857143 0.44285714 0.45714286 0.47142857 0.48571429 0.5 0.51428571 0.52857143 0.54285714 0.55714286 0.57142857 0.58571429 0.6 0.61428571 0.62857143 0.64285714 0.65714286 0.67142857 0.68571429 0.7 0.71428571 0.72857143 0.74285714 0.75714286 0.77142857 0.78571429 0.8 0.81428571 0.82857143 0.84285714 0.85714286 0.87142857 0.88571429 0.9 0.91428571 0.92857143 0.94285714 0.95714286 0.97142857 0.98571429 1 1 1 1 1 1
  arc A22 (4.8603, 10.5327) -> (4.3259, 10.7632) centre (0, 0) ccw
  spline S11 degree 5 poles (4.3259, 10.7632) (4.3223, 10.7603) (4.315, 10.7543) (4.3042, 10.7455) (4.2898, 10.7336) (4.2719, 10.7187) (4.254, 10.7038) (4.2363, 10.6888) (4.2187, 10.6737) (4.2011, 10.6586) (4.1836, 10.6434) (4.1663, 10.6282) (4.149, 10.6129) (4.1318, 10.5976) (4.1147, 10.5822) (4.0977, 10.5668) (4.0808, 10.5513) (4.064, 10.5357) (4.0472, 10.5201) (4.0306, 10.5045) (4.0141, 10.4887) (3.9977, 10.473) (3.9813, 10.4571) (3.9651, 10.4413) (3.949, 10.4253) (3.933, 10.4093) (3.917, 10.3933) (3.9012, 10.3772) (3.8855, 10.361) (3.8699, 10.3448) (3.8544, 10.3285) (3.839, 10.3122) (3.8237, 10.2958) (3.8086, 10.2794) (3.7935, 10.2629) (3.7786, 10.2463) (3.7637, 10.2297) (3.749, 10.213) (3.7344, 10.1963) (3.7199, 10.1795) (3.7055, 10.1626) (3.6913, 10.1457) (3.6772, 10.1288) (3.6632, 10.1117) (3.6493, 10.0947) (3.6356, 10.0775) (3.622, 10.0603) (3.6085, 10.043) (3.5952, 10.0257) (3.582, 10.0083) (3.5689, 9.9909) (3.556, 9.9734) (3.5432, 9.9558) (3.5306, 9.9381) (3.5182, 9.9204) (3.5059, 9.9026) (3.4937, 9.8847) (3.4817, 9.8668) (3.4698, 9.8489) (3.4582, 9.8308) (3.4467, 9.8127) (3.4354, 9.7944) (3.4244, 9.7761) (3.4137, 9.7577) (3.4032, 9.7391) (3.3928, 9.7205) (3.3826, 9.7019) (3.3725, 9.6832) (3.3626, 9.6645) (3.3531, 9.6456) (3.344, 9.6265) (3.3374, 9.611) (3.3328, 9.5992) (3.3299, 9.5913) (3.3285, 9.5873) knots -1 -1 -1 -1 -1 -1 -0.98571429 -0.97142857 -0.95714286 -0.94285714 -0.92857143 -0.91428571 -0.9 -0.88571429 -0.87142857 -0.85714286 -0.84285714 -0.82857143 -0.81428571 -0.8 -0.78571429 -0.77142857 -0.75714286 -0.74285714 -0.72857143 -0.71428571 -0.7 -0.68571429 -0.67142857 -0.65714286 -0.64285714 -0.62857143 -0.61428571 -0.6 -0.58571429 -0.57142857 -0.55714286 -0.54285714 -0.52857143 -0.51428571 -0.5 -0.48571429 -0.47142857 -0.45714286 -0.44285714 -0.42857143 -0.41428571 -0.4 -0.38571429 -0.37142857 -0.35714286 -0.34285714 -0.32857143 -0.31428571 -0.3 -0.28571429 -0.27142857 -0.25714286 -0.24285714 -0.22857143 -0.21428571 -0.2 -0.18571429 -0.17142857 -0.15714286 -0.14285714 -0.12857143 -0.11428571 -0.1 -0.08571429 -0.07142857 -0.05714286 -0.04285714 -0.02857143 -0.01428571 0 0 0 0 0 0
  line L11 (3.3285, 9.5873) -> (3.2427, 9.3417)
  arc A23 (3.1165, 9.2799) -> (3.2427, 9.3417) centre (3.1483, 9.3747) ccw
  arc A24 (3.1165, 9.2799) -> (2.4956, 9.4658) centre (0, 0) ccw
  arc A25 (2.4241, 9.5868) -> (2.4956, 9.4658) centre (2.5211, 9.5624) ccw
  line L12 (2.4241, 9.5868) -> (2.4874, 9.8391)
  spline S12 degree 5 poles (2.4874, 9.8391) (2.4884, 9.8432) (2.4903, 9.8514) (2.493, 9.8638) (2.496, 9.8804) (2.4989, 9.9013) (2.5013, 9.9223) (2.5033, 9.9434) (2.5052, 9.9646) (2.5069, 9.9858) (2.5084, 10.007) (2.5098, 10.0283) (2.511, 10.0496) (2.5119, 10.0709) (2.5125, 10.0923) (2.5129, 10.1138) (2.513, 10.1353) (2.513, 10.1568) (2.5128, 10.1784) (2.5124, 10.2) (2.5119, 10.2216) (2.5113, 10.2433) (2.5105, 10.265) (2.5095, 10.2867) (2.5083, 10.3084) (2.507, 10.3302) (2.5055, 10.3519) (2.5039, 10.3738) (2.5021, 10.3956) (2.5002, 10.4174) (2.4981, 10.4393) (2.4959, 10.4612) (2.4936, 10.4831) (2.4911, 10.505) (2.4885, 10.527) (2.4858, 10.549) (2.4829, 10.571) (2.4799, 10.593) (2.4768, 10.615) (2.4735, 10.637) (2.4701, 10.6591) (2.4666, 10.6811) (2.463, 10.7032) (2.4592, 10.7253) (2.4553, 10.7474) (2.4513, 10.7695) (2.4472, 10.7916) (2.4429, 10.8138) (2.4386, 10.8359) (2.4341, 10.8581) (2.4295, 10.8802) (2.4248, 10.9024) (2.4199, 10.9246) (2.415, 10.9468) (2.4099, 10.969) (2.4048, 10.9912) (2.3995, 11.0134) (2.3941, 11.0356) (2.3886, 11.0579) (2.383, 11.0801) (2.3773, 11.1024) (2.3714, 11.1246) (2.3655, 11.1469) (2.3594, 11.1691) (2.3533, 11.1914) (2.347, 11.2137) (2.3407, 11.2359) (2.3342, 11.2582) (2.3276, 11.2805) (2.3209, 11.3028) (2.3141, 11.3251) (2.3086, 11.3429) (2.3045, 11.3563) (2.3017, 11.3652) (2.3002, 11.3696) knots 0 0 0 0 0 0 0.01428571 0.02857143 0.04285714 0.05714286 0.07142857 0.08571429 0.1 0.11428571 0.12857143 0.14285714 0.15714286 0.17142857 0.18571429 0.2 0.21428571 0.22857143 0.24285714 0.25714286 0.27142857 0.28571429 0.3 0.31428571 0.32857143 0.34285714 0.35714286 0.37142857 0.38571429 0.4 0.41428571 0.42857143 0.44285714 0.45714286 0.47142857 0.48571429 0.5 0.51428571 0.52857143 0.54285714 0.55714286 0.57142857 0.58571429 0.6 0.61428571 0.62857143 0.64285714 0.65714286 0.67142857 0.68571429 0.7 0.71428571 0.72857143 0.74285714 0.75714286 0.77142857 0.78571429 0.8 0.81428571 0.82857143 0.84285714 0.85714286 0.87142857 0.88571429 0.9 0.91428571 0.92857143 0.94285714 0.95714286 0.97142857 0.98571429 1 1 1 1 1 1
  arc A26 (2.3002, 11.3696) -> (1.7271, 11.4707) centre (0, 0) ccw
  spline S13 degree 5 poles (1.7271, 11.4707) (1.7243, 11.467) (1.7186, 11.4596) (1.7101, 11.4484) (1.6988, 11.4336) (1.6848, 11.4149) (1.6709, 11.3963) (1.6571, 11.3776) (1.6434, 11.3589) (1.6298, 11.3401) (1.6163, 11.3213) (1.6029, 11.3025) (1.5896, 11.2837) (1.5764, 11.2648) (1.5633, 11.2459) (1.5504, 11.2269) (1.5375, 11.208) (1.5247, 11.1889) (1.512, 11.1699) (1.4995, 11.1508) (1.487, 11.1317) (1.4747, 11.1126) (1.4624, 11.0934) (1.4503, 11.0742) (1.4383, 11.055) (1.4264, 11.0357) (1.4146, 11.0165) (1.4029, 10.9971) (1.3914, 10.9778) (1.3799, 10.9584) (1.3686, 10.939) (1.3574, 10.9196) (1.3463, 10.9001) (1.3353, 10.8806) (1.3245, 10.8611) (1.3137, 10.8415) (1.3031, 10.8219) (1.2927, 10.8023) (1.2823, 10.7827) (1.2721, 10.763) (1.262, 10.7433) (1.252, 10.7235) (1.2422, 10.7038) (1.2325, 10.684) (1.223, 10.6642) (1.2136, 10.6443) (1.2043, 10.6244) (1.1952, 10.6045) (1.1862, 10.5846) (1.1773, 10.5646) (1.1686, 10.5446) (1.1601, 10.5246) (1.1518, 10.5045) (1.1436, 10.4844) (1.1355, 10.4643) (1.1277, 10.4442) (1.12, 10.424) (1.1124, 10.4038) (1.105, 10.3836) (1.0978, 10.3633) (1.0908, 10.343) (1.0841, 10.3227) (1.0776, 10.3023) (1.0714, 10.2819) (1.0655, 10.2614) (1.0597, 10.241) (1.054, 10.2205) (1.0485, 10.2) (1.0432, 10.1794) (1.0383, 10.1589) (1.0339, 10.1382) (1.031, 10.1216) (1.0292, 10.1091) (1.0283, 10.1007) (1.0278, 10.0965) knots -1 -1 -1 -1 -1 -1 -0.98571429 -0.97142857 -0.95714286 -0.94285714 -0.92857143 -0.91428571 -0.9 -0.88571429 -0.87142857 -0.85714286 -0.84285714 -0.82857143 -0.81428571 -0.8 -0.78571429 -0.77142857 -0.75714286 -0.74285714 -0.72857143 -0.71428571 -0.7 -0.68571429 -0.67142857 -0.65714286 -0.64285714 -0.62857143 -0.61428571 -0.6 -0.58571429 -0.57142857 -0.55714286 -0.54285714 -0.52857143 -0.51428571 -0.5 -0.48571429 -0.47142857 -0.45714286 -0.44285714 -0.42857143 -0.41428571 -0.4 -0.38571429 -0.37142857 -0.35714286 -0.34285714 -0.32857143 -0.31428571 -0.3 -0.28571429 -0.27142857 -0.25714286 -0.24285714 -0.22857143 -0.21428571 -0.2 -0.18571429 -0.17142857 -0.15714286 -0.14285714 -0.12857143 -0.11428571 -0.1 -0.08571429 -0.07142857 -0.05714286 -0.04285714 -0.02857143 -0.01428571 0 0 0 0 0 0
  line L13 (1.0278, 10.0965) -> (1.001, 9.8377)
  arc A27 (0.8924, 9.7484) -> (1.001, 9.8377) centre (0.9015, 9.848) ccw
  arc A28 (0.8924, 9.7484) -> (0.2454, 9.7861) centre (0, 0) ccw
  arc A29 (0.1479, 9.8874) -> (0.2454, 9.7861) centre (0.2479, 9.8861) ccw
  line L14 (0.1479, 9.8874) -> (0.1513, 10.1476)
  spline S14 degree 5 poles (0.1513, 10.1476) (0.1513, 10.1518) (0.1513, 10.1602) (0.151, 10.1728) (0.1501, 10.1897) (0.1481, 10.2107) (0.1456, 10.2317) (0.1427, 10.2527) (0.1396, 10.2737) (0.1364, 10.2947) (0.133, 10.3157) (0.1295, 10.3368) (0.1257, 10.3578) (0.1216, 10.3787) (0.1173, 10.3997) (0.1127, 10.4207) (0.1079, 10.4416) (0.1029, 10.4626) (0.0978, 10.4835) (0.0924, 10.5045) (0.087, 10.5254) (0.0813, 10.5463) (0.0755, 10.5672) (0.0696, 10.5881) (0.0634, 10.609) (0.0571, 10.6299) (0.0506, 10.6507) (0.044, 10.6716) (0.0373, 10.6924) (0.0304, 10.7132) (0.0233, 10.734) (0.0161, 10.7548) (0.0088, 10.7756) (0.0014, 10.7964) (-0.0062, 10.8171) (-0.014, 10.8379) (-0.0219, 10.8586) (-0.0299, 10.8793) (-0.038, 10.9) (-0.0462, 10.9207) (-0.0546, 10.9414) (-0.0631, 10.962) (-0.0718, 10.9827) (-0.0805, 11.0033) (-0.0894, 11.0239) (-0.0984, 11.0445) (-0.1075, 11.0651) (-0.1168, 11.0856) (-0.1261, 11.1062) (-0.1356, 11.1267) (-0.1452, 11.1472) (-0.1549, 11.1677) (-0.1647, 11.1882) (-0.1746, 11.2087) (-0.1847, 11.2291) (-0.1948, 11.2495) (-0.2051, 11.2699) (-0.2154, 11.2903) (-0.2259, 11.3107) (-0.2365, 11.331) (-0.2472, 11.3513) (-0.258, 11.3716) (-0.2689, 11.3919) (-0.2799, 11.4122) (-0.2911, 11.4324) (-0.3023, 11.4527) (-0.3136, 11.4729) (-0.3251, 11.4931) (-0.3366, 11.5132) (-0.3482, 11.5334) (-0.36, 11.5535) (-0.3694, 11.5696) (-0.3766, 11.5816) (-0.3814, 11.5896) (-0.3838, 11.5936) knots 0 0 0 0 0 0 0.01428571 0.02857143 0.04285714 0.05714286 0.07142857 0.08571429 0.1 0.11428571 0.12857143 0.14285714 0.15714286 0.17142857 0.18571429 0.2 0.21428571 0.22857143 0.24285714 0.25714286 0.27142857 0.28571429 0.3 0.31428571 0.32857143 0.34285714 0.35714286 0.37142857 0.38571429 0.4 0.41428571 0.42857143 0.44285714 0.45714286 0.47142857 0.48571429 0.5 0.51428571 0.52857143 0.54285714 0.55714286 0.57142857 0.58571429 0.6 0.61428571 0.62857143 0.64285714 0.65714286 0.67142857 0.68571429 0.7 0.71428571 0.72857143 0.74285714 0.75714286 0.77142857 0.78571429 0.8 0.81428571 0.82857143 0.84285714 0.85714286 0.87142857 0.88571429 0.9 0.91428571 0.92857143 0.94285714 0.95714286 0.97142857 0.98571429 1 1 1 1 1 1
  arc A30 (-0.3838, 11.5936) -> (-0.9648, 11.5598) centre (0, 0) ccw
  spline S15 degree 5 poles (-0.9648, 11.5598) (-0.9667, 11.5555) (-0.9705, 11.547) (-0.9762, 11.5342) (-0.9837, 11.5171) (-0.9931, 11.4958) (-1.0023, 11.4744) (-1.0114, 11.4531) (-1.0204, 11.4317) (-1.0293, 11.4103) (-1.0381, 11.3889) (-1.0468, 11.3675) (-1.0554, 11.3461) (-1.0639, 11.3247) (-1.0723, 11.3033) (-1.0805, 11.2818) (-1.0887, 11.2604) (-1.0967, 11.239) (-1.1047, 11.2175) (-1.1125, 11.1961) (-1.1202, 11.1746) (-1.1278, 11.1531) (-1.1353, 11.1317) (-1.1427, 11.1102) (-1.1499, 11.0887) (-1.1571, 11.0672) (-1.1641, 11.0457) (-1.171, 11.0242) (-1.1778, 11.0027) (-1.1845, 10.9813) (-1.191, 10.9598) (-1.1974, 10.9383) (-1.2037, 10.9168) (-1.2099, 10.8952) (-1.216, 10.8737) (-1.2219, 10.8522) (-1.2277, 10.8307) (-1.2334, 10.8092) (-1.2389, 10.7877) (-1.2443, 10.7662) (-1.2496, 10.7447) (-1.2547, 10.7232) (-1.2597, 10.7017) (-1.2646, 10.6802) (-1.2693, 10.6587) (-1.2739, 10.6373) (-1.2783, 10.6158) (-1.2826, 10.5943) (-1.2868, 10.5728) (-1.2908, 10.5514) (-1.2946, 10.5299) (-1.2983, 10.5084) (-1.3018, 10.487) (-1.3051, 10.4656) (-1.3083, 10.4441) (-1.3113, 10.4227) (-1.3142, 10.4013) (-1.3169, 10.3799) (-1.3194, 10.3585) (-1.3217, 10.3371) (-1.3239, 10.3158) (-1.3257, 10.2944) (-1.3273, 10.2731) (-1.3286, 10.2518) (-1.3297, 10.2305) (-1.3306, 10.2093) (-1.3314, 10.188) (-1.332, 10.1668) (-1.3325, 10.1456) (-1.3325, 10.1245) (-1.332, 10.1034) (-1.331, 10.0865) (-1.3298, 10.0739) (-1.3288, 10.0656) (-1.3283, 10.0614) knots -1 -1 -1 -1 -1 -1 -0.98571429 -0.97142857 -0.95714286 -0.94285714 -0.92857143 -0.91428571 -0.9 -0.88571429 -0.87142857 -0.85714286 -0.84285714 -0.82857143 -0.81428571 -0.8 -0.78571429 -0.77142857 -0.75714286 -0.74285714 -0.72857143 -0.71428571 -0.7 -0.68571429 -0.67142857 -0.65714286 -0.64285714 -0.62857143 -0.61428571 -0.6 -0.58571429 -0.57142857 -0.55714286 -0.54285714 -0.52857143 -0.51428571 -0.5 -0.48571429 -0.47142857 -0.45714286 -0.44285714 -0.42857143 -0.41428571 -0.4 -0.38571429 -0.37142857 -0.35714286 -0.34285714 -0.32857143 -0.31428571 -0.3 -0.28571429 -0.27142857 -0.25714286 -0.24285714 -0.22857143 -0.21428571 -0.2 -0.18571429 -0.17142857 -0.15714286 -0.14285714 -0.12857143 -0.11428571 -0.1 -0.08571429 -0.07142857 -0.05714286 -0.04285714 -0.02857143 -0.01428571 0 0 0 0 0 0
  line L15 (-1.3283, 10.0614) -> (-1.2947, 9.8034)
  arc A31 (-1.3798, 9.6915) -> (-1.2947, 9.8034) centre (-1.3939, 9.7905) ccw
  arc A32 (-1.3798, 9.6915) -> (-2.0181, 9.5789) centre (0, 0) ccw
  arc A33 (-2.1363, 9.655) -> (-2.0181, 9.5789) centre (-2.0387, 9.6768) ccw
  line L16 (-2.1363, 9.655) -> (-2.193, 9.9089)
  spline S16 degree 5 poles (-2.193, 9.9089) (-2.1939, 9.913) (-2.1959, 9.9212) (-2.1991, 9.9335) (-2.2039, 9.9496) (-2.2106, 9.9696) (-2.2179, 9.9895) (-2.2256, 10.0093) (-2.2334, 10.029) (-2.2414, 10.0487) (-2.2495, 10.0684) (-2.2578, 10.088) (-2.2664, 10.1075) (-2.2751, 10.127) (-2.2842, 10.1465) (-2.2935, 10.1658) (-2.303, 10.1851) (-2.3127, 10.2043) (-2.3226, 10.2235) (-2.3326, 10.2426) (-2.3427, 10.2617) (-2.353, 10.2808) (-2.3635, 10.2998) (-2.3741, 10.3187) (-2.3849, 10.3376) (-2.3958, 10.3565) (-2.4069, 10.3753) (-2.4182, 10.3941) (-2.4296, 10.4128) (-2.4411, 10.4314) (-2.4527, 10.4501) (-2.4645, 10.4686) (-2.4764, 10.4872) (-2.4885, 10.5057) (-2.5007, 10.5241) (-2.513, 10.5425) (-2.5254, 10.5609) (-2.538, 10.5792) (-2.5507, 10.5975) (-2.5635, 10.6157) (-2.5764, 10.6339) (-2.5894, 10.652) (-2.6026, 10.6701) (-2.6159, 10.6881) (-2.6293, 10.7061) (-2.6428, 10.7241) (-2.6564, 10.742) (-2.6701, 10.7599) (-2.684, 10.7777) (-2.6979, 10.7955) (-2.712, 10.8133) (-2.7261, 10.831) (-2.7404, 10.8486) (-2.7548, 10.8663) (-2.7693, 10.8838) (-2.7839, 10.9014) (-2.7986, 10.9188) (-2.8134, 10.9363) (-2.8282, 10.9537) (-2.8432, 10.971) (-2.8583, 10.9883) (-2.8735, 11.0056) (-2.8888, 11.0228) (-2.9042, 11.04) (-2.9197, 11.0572) (-2.9353, 11.0742) (-2.951, 11.0913) (-2.9668, 11.1083) (-2.9826, 11.1253) (-2.9986, 11.1422) (-3.0147, 11.159) (-3.0276, 11.1725) (-3.0373, 11.1826) (-3.0439, 11.1893) (-3.0471, 11.1926) knots 0 0 0 0 0 0 0.01428571 0.02857143 0.04285714 0.05714286 0.07142857 0.08571429 0.1 0.11428571 0.12857143 0.14285714 0.15714286 0.17142857 0.18571429 0.2 0.21428571 0.22857143 0.24285714 0.25714286 0.27142857 0.28571429 0.3 0.31428571 0.32857143 0.34285714 0.35714286 0.37142857 0.38571429 0.4 0.41428571 0.42857143 0.44285714 0.45714286 0.47142857 0.48571429 0.5 0.51428571 0.52857143 0.54285714 0.55714286 0.57142857 0.58571429 0.6 0.61428571 0.62857143 0.64285714 0.65714286 0.67142857 0.68571429 0.7 0.71428571 0.72857143 0.74285714 0.75714286 0.77142857 0.78571429 0.8 0.81428571 0.82857143 0.84285714 0.85714286 0.87142857 0.88571429 0.9 0.91428571 0.92857143 0.94285714 0.95714286 0.97142857 0.98571429 1 1 1 1 1 1
  arc A34 (-3.0471, 11.1926) -> (-3.6046, 11.0257) centre (0, 0) ccw
  spline S17 degree 5 poles (-3.6046, 11.0257) (-3.6055, 11.0211) (-3.6073, 11.012) (-3.6099, 10.9982) (-3.6133, 10.9798) (-3.6174, 10.9569) (-3.6215, 10.934) (-3.6254, 10.9111) (-3.6292, 10.8882) (-3.633, 10.8654) (-3.6366, 10.8425) (-3.6401, 10.8197) (-3.6436, 10.7969) (-3.6469, 10.7741) (-3.6501, 10.7513) (-3.6532, 10.7286) (-3.6562, 10.7058) (-3.6591, 10.6831) (-3.6618, 10.6604) (-3.6645, 10.6377) (-3.6671, 10.615) (-3.6695, 10.5924) (-3.6718, 10.5698) (-3.6741, 10.5472) (-3.6762, 10.5246) (-3.6782, 10.5021) (-3.68, 10.4795) (-3.6818, 10.457) (-3.6835, 10.4346) (-3.685, 10.4121) (-3.6864, 10.3897) (-3.6877, 10.3673) (-3.6889, 10.3449) (-3.6899, 10.3225) (-3.6908, 10.3002) (-3.6917, 10.2779) (-3.6923, 10.2557) (-3.6929, 10.2334) (-3.6933, 10.2112) (-3.6936, 10.1891) (-3.6938, 10.1669) (-3.6939, 10.1448) (-3.6938, 10.1227) (-3.6935, 10.1007) (-3.6932, 10.0787) (-3.6927, 10.0567) (-3.692, 10.0348) (-3.6913, 10.0129) (-3.6904, 9.9911) (-3.6893, 9.9693) (-3.6881, 9.9475) (-3.6867, 9.9258) (-3.6852, 9.9041) (-3.6835, 9.8825) (-3.6816, 9.8609) (-3.6796, 9.8394) (-3.6774, 9.8179) (-3.6751, 9.7964) (-3.6727, 9.775) (-3.67, 9.7537) (-3.6672, 9.7324) (-3.664, 9.7112) (-3.6607, 9.6901) (-3.657, 9.6691) (-3.6532, 9.6481) (-3.6492, 9.6272) (-3.645, 9.6064) (-3.6408, 9.5856) (-3.6363, 9.5649) (-3.6315, 9.5443) (-3.6261, 9.5238) (-3.6212, 9.5077) (-3.6172, 9.4957) (-3.6143, 9.4878) (-3.6128, 9.4838) knots -1 -1 -1 -1 -1 -1 -0.98571429 -0.97142857 -0.95714286 -0.94285714 -0.92857143 -0.91428571 -0.9 -0.88571429 -0.87142857 -0.85714286 -0.84285714 -0.82857143 -0.81428571 -0.8 -0.78571429 -0.77142857 -0.75714286 -0.74285714 -0.72857143 -0.71428571 -0.7 -0.68571429 -0.67142857 -0.65714286 -0.64285714 -0.62857143 -0.61428571 -0.6 -0.58571429 -0.57142857 -0.55714286 -0.54285714 -0.52857143 -0.51428571 -0.5 -0.48571429 -0.47142857 -0.45714286 -0.44285714 -0.42857143 -0.41428571 -0.4 -0.38571429 -0.37142857 -0.35714286 -0.34285714 -0.32857143 -0.31428571 -0.3 -0.28571429 -0.27142857 -0.25714286 -0.24285714 -0.22857143 -0.21428571 -0.2 -0.18571429 -0.17142857 -0.15714286 -0.14285714 -0.12857143 -0.11428571 -0.1 -0.08571429 -0.07142857 -0.05714286 -0.04285714 -0.02857143 -0.01428571 0 0 0 0 0 0
  line L17 (-3.6128, 9.4838) -> (-3.5207, 9.2405)
  arc A35 (-3.5776, 9.112) -> (-3.5207, 9.2405) centre (-3.6142, 9.2051) ccw
  arc A36 (-3.5776, 9.112) -> (-4.1727, 8.8553) centre (0, 0) ccw
  arc A37 (-4.3053, 8.9021) -> (-4.1727, 8.8553) centre (-4.2154, 8.9458) ccw
  line L18 (-4.3053, 8.9021) -> (-4.419, 9.1361)